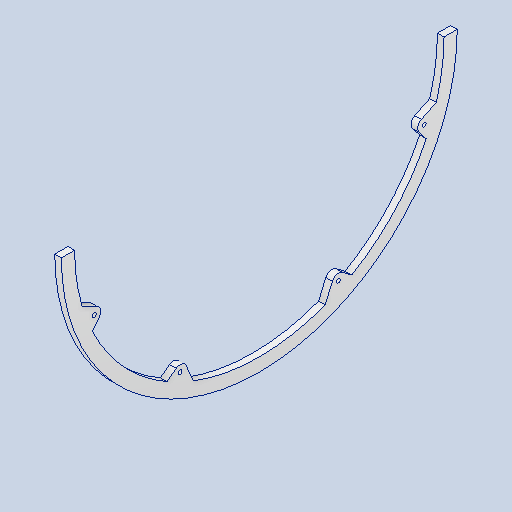
# Autodesk Inventor part: base_weel-v2-Plate-2
Saved by Autodesk Inventor 2025.2 (Build 292293000, 293)
## iProperties
Created: 2025-01-06
Part Number: base_weel-v2-Plate-2
Material: アルミニウム 6061
Document SubType Name: Modeling
Designer: haruy
Density: 2.7 g/cm^3
Appearance: アルミニウム - フラット
Author: haruy
Autodesk Inventor part; units mm, degrees
ref_plane "YZ Plane" through (0, 0, 0) normal (1, 0, 0) x (0, 1, 0)
ref_plane "XZ Plane" through (0, 0, 0) normal (0, 1, 0) x (-1, 0, 0)
ref_plane "XY Plane" through (0, 0, 0) normal (0, 0, 1) x (1, 0, 0)
derived "base_weel-v2-Sketch-Base.ipt"
sketch "スケッチ1" plane through (0, 0, 0) normal (1, 0, 0) x (0, 1, 0)
  line L0 (-315, 315) -> (315, 315)
  line L1 (315, 315) -> (315, -315)
  line L2 (315, -315) -> (-315, -315)
  line L3 (-315, -315) -> (-315, 315)
  line L4 (-315, 315) -> (315, -315) construction
  line L5 (315, 315) -> (-315, -315) construction
  line L6 (-315, 210) -> (-300, 210)
  line L7 (-300, 210) -> (-300, -210)
  line L8 (-300, -210) -> (-315, -210)
  line L9 (-315, -210) -> (-315, 210)
  line L10 (242, 315) -> (-242, 315)
  line L11 (-242, 315) -> (-242, 295)
  line L12 (-242, 295) -> (242, 295)
  line L13 (242, 295) -> (242, 315)
  line L14 (-300, 210) -> (-300, 315)
  line L15 (0, 0) -> (-956.5973, 0)
  circle A0 centre (0, 0) radius 400
  line L16 (-330, 25) -> (-380, 25)
  line L17 (-380, 25) -> (-380, -25)
  line L18 (-380, -25) -> (-330, -25)
  line L19 (-330, -25) -> (-330, 25)
  line L20 (0, 0) -> (0, -630.9179)
  line L21 (-315, 40) -> (-395, 40)
  line L22 (-395, 40) -> (-395, 30)
  line L23 (-395, 30) -> (-315, 30)
  line L24 (-315, 30) -> (-315, 40)
  line L25 (-395, 30) -> (-385, 30)
  line L26 (-385, 30) -> (-385, 0)
  line L27 (-385, 0) -> (-395, 0)
  line L28 (-395, 0) -> (-395, 30)
  line L29 (300, 210) -> (315, 210)
  line L30 (315, 210) -> (315, -210)
  line L31 (315, -210) -> (300, -210)
  line L32 (300, -210) -> (300, 210)
  line L33 (-222.2183, -315) -> (242, -315)
  line L34 (242, -315) -> (242, -295)
  line L35 (242, -295) -> (-242, -295)
  line L36 (315, 315) -> (0, 0)
  line L37 (315, 125) -> (315, 145)
  circle A1 centre (512, 0) radius 122.5
  circle A2 centre (179.6905, 0) radius 600
  circle A3 centre (541.6815, 0) radius 200
  circle A4 centre (0, 0) radius 10
  arc A5 (0, 150) -> (0, -150) centre (0, 0) ccw
  arc A6 (0, 140) -> (0, -140) centre (0, 0) ccw
  line L38 (-146.3272, 32.9904) -> (-136.572, 30.791) construction
  line L39 (-137.5812, 37.6817) -> (-140.4404, 25)
  line L40 (-140.4404, 25) -> (-145.318, 26.0997)
  line L41 (-145.318, 26.0997) -> (-142.4588, 38.7814)
  line L42 (-142.4588, 38.7814) -> (-137.5812, 37.6817)
  arc A7 (-29.1302, 142.0438) -> (-29.1302, -142.0438) centre (0, 0) ccw construction
  circle A8 centre (-151.4904, 39.2799) radius 6.5
  circle A9 centre (-129.0401, 34.2184) radius 6.5 construction
  circle A10 centre (-129.0401, 34.2184) radius 1.5 construction
  circle A11 centre (-151.4904, 39.2799) radius 1.5
  line L43 (-104.1709, 22.5) -> (-174.1362, 22.5) construction
  line L44 (-174.1362, 22.5) -> (-174.1362, 7.5)
  line L45 (-174.1362, 7.5) -> (-104.1709, 7.5) construction
  line L46 (-104.1709, 7.5) -> (-104.1709, 22.5)
  circle A12 centre (-129.0401, -34.2184) radius 6.5 construction
  circle A13 centre (-129.0401, -34.2184) radius 1.5 construction
  line L47 (-142.4588, -38.7814) -> (-137.5812, -37.6817)
  line L48 (-145.318, -26.0997) -> (-142.4588, -38.7814)
  line L49 (-137.5812, -37.6817) -> (-140.4404, -25)
  line L50 (-140.4404, -25) -> (-145.318, -26.0997)
  circle A14 centre (-151.4904, -39.2799) radius 6.5
  circle A15 centre (-151.4904, -39.2799) radius 1.5
  line L51 (-146.3272, -32.9904) -> (-136.572, -30.791) construction
  line L52 (-104.1709, -22.5) -> (-174.1362, -22.5) construction
  line L53 (-174.1362, -7.5) -> (-104.1709, -7.5) construction
  line L54 (-104.1709, -7.5) -> (-104.1709, -22.5)
  line L55 (-174.1362, -22.5) -> (-174.1362, -7.5)
  line L56 (-151.4904, 39.2799) -> (-129.0401, 34.2184) construction
  line L57 (-129.0401, 34.2184) -> (-129.59, 31.7796) construction
  line L58 (-129.59, 31.7796) -> (-152.0402, 36.8412) construction
  line L59 (-152.0402, 36.8412) -> (-151.4904, 39.2799) construction
  line L60 (-129.0401, 34.2184) -> (-151.4904, 39.2799) construction
  line L61 (-151.4904, 39.2799) -> (-150.9405, 41.7187) construction
  line L62 (-150.9405, 41.7187) -> (-128.4903, 36.6572) construction
  line L63 (-128.4903, 36.6572) -> (-129.0401, 34.2184) construction
  line L64 (-128.4903, 36.6572) -> (-129.59, 31.7796) construction
  line L65 (-129.59, 31.7796) -> (-117.8838, 29.1404) construction
  line L66 (-117.8838, 29.1404) -> (-116.7841, 34.0179) construction
  line L67 (-116.7841, 34.0179) -> (-128.4903, 36.6572) construction
  line L68 (-150.9405, 41.7187) -> (-152.0402, 36.8412) construction
  line L69 (-152.0402, 36.8412) -> (-163.7464, 39.4804) construction
  line L70 (-163.7464, 39.4804) -> (-162.6467, 44.358) construction
  line L71 (-162.6467, 44.358) -> (-150.9405, 41.7187) construction
  line L72 (-155.2683, 45.2572) -> (-128.9412, 39.3216) construction
  line L73 (-128.9412, 39.3216) -> (-132.2403, 24.6889)
  line L74 (-132.2403, 24.6889) -> (-158.5673, 30.6245) construction
  line L75 (-158.5673, 30.6245) -> (-155.2683, 45.2572)
  line L76 (-128.9412, -39.3216) -> (-132.2403, -24.6889)
  line L77 (-155.2683, -45.2572) -> (-128.9412, -39.3216)
  line L78 (-132.2403, -24.6889) -> (-158.5673, -30.6245) construction
  line L79 (-158.5673, -30.6245) -> (-155.2683, -45.2572)
  arc A16 (-132.2403, 24.6889) -> (-132.2403, -24.6889) centre (0, 0) ccw
  arc A17 (-158.5673, 30.6245) -> (-158.5673, -30.6245) centre (0, 0) ccw
  circle A18 centre (-152.5, 15) radius 1.25
  line L80 (-145, 0) -> (-145, 74.7382) construction
  circle A19 centre (-137.5, 15) radius 1.25
  circle A20 centre (-137.5, -15) radius 1.25
  circle A21 centre (-152.5, -15) radius 1.25
  line L81 (0, 0) -> (0, 140)
  line L82 (0, 0) -> (-47.8828, 131.557) construction
  line L83 (0, 140) -> (0, 150)
  line L84 (-137.5846, 25.8938) -> (-134.2855, 40.5265)
  line L85 (-137.5846, -25.8938) -> (-134.2855, -40.5265)
  circle A22 centre (0, 0) radius 20
  line L86 (300, 70) -> (-300, 70)
  line L87 (-300, 70) -> (-300, 50)
  line L88 (-300, 50) -> (300, 50)
  line L89 (300, 50) -> (300, 70)
  line L90 (-40, 295) -> (-60, 295)
  line L91 (-60, 295) -> (-60, 70)
  line L92 (-60, 70) -> (-40, 70)
  line L93 (-40, 70) -> (-40, 295)
  line L94 (-60, -295) -> (-60, -70) construction
  line L95 (-40, -70) -> (-40, -295) construction
  line L96 (300, -70) -> (-300, -70) construction
  line L97 (-300, -50) -> (300, -50) construction
  line L98 (-40, 70) -> (-40, -70)
  line L99 (40, 70) -> (40, -70)
  circle A23 centre (20, 60) radius 1.5
  circle A24 centre (-20, 60) radius 1.5
  circle A25 centre (-20, -60) radius 1.5
  circle A26 centre (20, -60) radius 1.5
  circle A27 centre (-50, 125) radius 1.5
  circle A28 centre (-50, 125) radius 5
  circle A29 centre (-120, 60) radius 5
  circle A30 centre (-120, 60) radius 1.5
  line L100 (-40, 134.1641) -> (-45.5009, 122.8186)
  line L101 (-53.0865, 121.0664) -> (-60, 126.4911)
  line L102 (-130.767, 50) -> (-118.047, 55.3972)
  line L103 (-121.2436, 70) -> (-115.9982, 62.9976)
  line L104 (-40, -134.1641) -> (-45.5009, -122.8186)
  circle A31 centre (-50, -125) radius 5
  circle A32 centre (-50, -125) radius 1.5
  line L105 (-53.0865, -121.0664) -> (-60, -126.4911)
  line L106 (-121.2436, -70) -> (-115.9982, -62.9976)
  circle A33 centre (-120, -60) radius 5
  circle A34 centre (-120, -60) radius 1.5
  line L107 (-130.767, -50) -> (-118.047, -55.3972)
  line L108 (-242, -295) -> (-242, -315)
  line L109 (242, 315) -> (222, 315)
  line L110 (222, 315) -> (222, 295)
  line L111 (222, 295) -> (242, 295)
  line L112 (242, 295) -> (242, 315)
  line L113 (242, -315) -> (222, -315)
  line L114 (222, -315) -> (222, -295)
  line L115 (222, -295) -> (242, -295)
  line L116 (242, -295) -> (242, -315)
  line L117 (212, 295) -> (300, 207)
  line L118 (300, 207) -> (289.3934, 196.3934)
  line L119 (289.3934, 196.3934) -> (201.3934, 284.3934)
  line L120 (201.3934, 284.3934) -> (212, 295)
  line L121 (212, 295) -> (212, 315)
  line L122 (213.5485, 293.4515) -> (202.9419, 282.8449)
  line L123 (205.7703, 280.0165) -> (280.0165, 205.7703)
  line L124 (280.0165, 205.7703) -> (239.0043, 164.7581)
  line L125 (239.0043, 164.7581) -> (164.7581, 239.0043)
  line L126 (164.7581, 239.0043) -> (205.7703, 280.0165)
  line L127 (298.4013, 208.5987) -> (287.7947, 197.9921)
  line L128 (111.018, 292.7444) -> (296.9871, 106.7753)
  line L129 (296.9871, 106.7753) -> (286.3805, 96.1687)
  line L130 (286.3805, 96.1687) -> (100.4114, 282.1378)
  line L131 (100.4114, 282.1378) -> (111.018, 292.7444)
  line L132 (221.6802, 285.3198) -> (211.0736, 274.7132)
  line L133 (285.3198, 221.6802) -> (274.7132, 211.0736)
  circle A35 centre (211.7807, 284.6127) radius 1.5
  circle A36 centre (222.3873, 274.0061) radius 1.5
  circle A37 centre (289.5624, 206.831) radius 1.5
  circle A38 centre (275.4203, 220.9731) radius 1.5
  circle A39 centre (112.7858, 280.3701) radius 1.5
  circle A40 centre (119.8568, 273.299) radius 1.5
  circle A41 centre (284.6127, 108.5431) radius 1.5
  circle A42 centre (277.5416, 115.6142) radius 1.5
  line L134 (201.3934, 284.3934) -> (190.7868, 295)
  circle A43 centre (202, 305) radius 1.5
  circle A44 centre (192, 305) radius 1.5
  line L135 (187, 315) -> (187, 295)
  line L136 (111.018, 292.7444) -> (108.7624, 295)
  line L137 (108.7624, 295) -> (108.7624, 315)
  line L138 (100.4114, 282.1378) -> (87.5492, 295)
  circle A45 centre (98.7624, 305) radius 1.5
  circle A46 centre (88.7624, 305) radius 1.5
  line L139 (83.7624, 315) -> (83.7624, 295)
  circle A47 centre (307.5, 197) radius 1.5
  circle A48 centre (307.5, 187) radius 1.5
  line L140 (289.3934, 196.3934) -> (300, 185.7868)
  line L141 (300, 207) -> (315, 207)
  line L142 (315, 182) -> (300, 182)
  line L143 (296.9871, 106.7753) -> (300, 103.7624)
  line L144 (286.3805, 96.1687) -> (300, 82.5492)
  line L145 (300, 103.7624) -> (315, 103.7624)
  circle A49 centre (307.5, 93.7624) radius 1.5
  circle A50 centre (307.5, 83.7624) radius 1.5
  line L146 (300, 78.7624) -> (315, 78.7624)
  line L147 (-212, 295) -> (-212, 315)
  circle A51 centre (-202, 305) radius 1.5
  circle A52 centre (-192, 305) radius 1.5
  line L148 (-187, 315) -> (-187, 295)
  line L149 (-108.7624, 295) -> (-108.7624, 315)
  circle A53 centre (-98.7624, 305) radius 1.5
  circle A54 centre (-88.7624, 305) radius 1.5
  line L150 (-83.7624, 315) -> (-83.7624, 295)
  line L151 (-100.4114, 282.1378) -> (-87.5492, 295)
  line L152 (-111.018, 292.7444) -> (-108.7624, 295)
  line L153 (-111.018, 292.7444) -> (-296.9871, 106.7753)
  line L154 (-100.4114, 282.1378) -> (-111.018, 292.7444)
  line L155 (-286.3805, 96.1687) -> (-100.4114, 282.1378)
  circle A55 centre (-112.7858, 280.3701) radius 1.5
  circle A56 centre (-119.8568, 273.299) radius 1.5
  line L156 (-296.9871, 106.7753) -> (-286.3805, 96.1687)
  line L157 (-296.9871, 106.7753) -> (-300, 103.7624)
  line L158 (-286.3805, 96.1687) -> (-300, 82.5492)
  line L159 (-300, 78.7624) -> (-315, 78.7624)
  line L160 (-300, 103.7624) -> (-315, 103.7624)
  circle A57 centre (-307.5, 93.7624) radius 1.5
  circle A58 centre (-307.5, 83.7624) radius 1.5
  line L161 (-280.0165, 205.7703) -> (-239.0043, 164.7581)
  line L162 (-164.7581, 239.0043) -> (-205.7703, 280.0165)
  line L163 (-289.3934, 196.3934) -> (-201.3934, 284.3934)
  line L164 (-201.3934, 284.3934) -> (-190.7868, 295)
  line L165 (-212, 295) -> (-300, 207)
  line L166 (-213.5485, 293.4515) -> (-202.9419, 282.8449)
  line L167 (-221.6802, 285.3198) -> (-211.0736, 274.7132)
  circle A59 centre (-275.4203, 220.9731) radius 1.5
  circle A60 centre (-289.5624, 206.831) radius 1.5
  line L168 (-298.4013, 208.5987) -> (-287.7947, 197.9921)
  line L169 (-289.3934, 196.3934) -> (-300, 185.7868)
  line L170 (-300, 207) -> (-315, 207)
  circle A61 centre (-307.5, 197) radius 1.5
  circle A62 centre (-307.5, 187) radius 1.5
  line L171 (-315, 182) -> (-300, 182)
  circle A63 centre (-275.4203, 220.9731) radius 1.5
  circle A64 centre (-289.5624, 206.831) radius 1.5
  circle A65 centre (-211.7807, 284.6127) radius 1.5
  circle A66 centre (-222.3873, 274.0061) radius 1.5
  circle A67 centre (-307.5, -93.7624) radius 1.5
  circle A68 centre (-307.5, -83.7624) radius 1.5
  circle A69 centre (-307.5, -187) radius 1.5
  circle A70 centre (-307.5, -197) radius 1.5
  line L172 (-111.018, -292.7444) -> (-296.9871, -106.7753)
  line L173 (-286.3805, -96.1687) -> (-100.4114, -282.1378)
  line L174 (-296.9871, -106.7753) -> (-286.3805, -96.1687)
  line L175 (-212, -295) -> (-300, -207)
  line L176 (-289.3934, -196.3934) -> (-201.3934, -284.3934)
  circle A71 centre (-289.5624, -206.831) radius 1.5
  circle A72 centre (-275.4203, -220.9731) radius 1.5
  line L177 (-298.4013, -208.5987) -> (-287.7947, -197.9921)
  circle A73 centre (-222.3873, -274.0061) radius 1.5
  line L178 (-221.6802, -285.3198) -> (-211.0736, -274.7132)
  line L179 (-213.5485, -293.4515) -> (-202.9419, -282.8449)
  circle A74 centre (-211.7807, -284.6127) radius 1.5
  circle A75 centre (-119.8568, -273.299) radius 1.5
  circle A76 centre (-112.7858, -280.3701) radius 1.5
  line L180 (-100.4114, -282.1378) -> (-111.018, -292.7444)
  circle A77 centre (-202, -305) radius 1.5
  circle A78 centre (-192, -305) radius 1.5
  circle A79 centre (-98.7624, -305) radius 1.5
  circle A80 centre (-88.7624, -305) radius 1.5
  circle A81 centre (98.7624, -305) radius 1.5
  circle A82 centre (88.7624, -305) radius 1.5
  line L181 (286.3805, -96.1687) -> (100.4114, -282.1378)
  line L182 (100.4114, -282.1378) -> (111.018, -292.7444)
  line L183 (111.018, -292.7444) -> (296.9871, -106.7753)
  circle A83 centre (112.7858, -280.3701) radius 1.5
  circle A84 centre (119.8568, -273.299) radius 1.5
  circle A85 centre (192, -305) radius 1.5
  circle A86 centre (202, -305) radius 1.5
  line L184 (289.3934, -196.3934) -> (201.3934, -284.3934)
  line L185 (213.5485, -293.4515) -> (202.9419, -282.8449)
  line L186 (212, -295) -> (300, -207)
  circle A87 centre (211.7807, -284.6127) radius 1.5
  circle A88 centre (222.3873, -274.0061) radius 1.5
  circle A89 centre (275.4203, -220.9731) radius 1.5
  circle A90 centre (289.5624, -206.831) radius 1.5
  line L187 (298.4013, -208.5987) -> (287.7947, -197.9921)
  circle A91 centre (307.5, -197) radius 1.5
  circle A92 centre (307.5, -187) radius 1.5
  line L188 (296.9871, -106.7753) -> (286.3805, -96.1687)
  circle A93 centre (284.6127, -108.5431) radius 1.5
  circle A94 centre (277.5416, -115.6142) radius 1.5
  circle A95 centre (307.5, -93.7624) radius 1.5
  circle A96 centre (307.5, -83.7624) radius 1.5
  circle A97 centre (-284.6127, 108.5431) radius 1.5
  circle A98 centre (-277.5416, 115.6142) radius 1.5
  circle A99 centre (-284.6127, -108.5431) radius 1.5
  circle A100 centre (-277.5416, -115.6142) radius 1.5
  line L189 (242, 295) -> (222, 295)
  line L190 (222, 295) -> (222, 243)
  line L191 (222, 243) -> (242, 243)
  line L192 (242, 243) -> (242, 295)
  point P0 (-141.4496, 31.8907)
  point P1 (-129.0401, 34.2184)
  point P2 (-150, 0)
  point P3 (0, -140)
  point P4 (-242, 305)
ref_plane "作業平面1" through (0, 0, 0) normal (1, 0, 0) x (0, 1, 0)
extrude "押し出し1" add sketch "スケッチ1" against normal blind 5 contours A5 L77 A6 L20 | L88 A6 L15 A5 | A5 L86 A6 L88 | L15 A6 L85 L77 A5 | A5 L91 A6 L86 | A6 L103 A29 L102 | A5 L93 A6 L91 | A6 L105 A31 L104 | L85 A6 L77 | A29 | A5 L83 A6 L93 | A6 L100 A28 L101 | A31 | A28 | A6 L107 A33 L106 | A33 | L39 L40 L41 L42 | L48 L50 L49 L47
